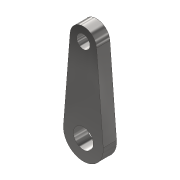
# Autodesk Inventor part: Eslabón 2
Saved by Autodesk Inventor 2021 (Build 250183000, 183)
## iProperties
Created: 2021-10-18
Part Number: Eslabón 2
Material: Stainless Steel
Document SubType Name: Modeling
Designer: Usuario
Density: 8 g/cm^3
Appearance: Semi-Polished
Author: Usuario
Autodesk Inventor part; units mm, degrees
ref_plane "YZ Plane" through (0, 0, 0) normal (1, 0, 0) x (0, 1, 0)
ref_plane "XZ Plane" through (0, 0, 0) normal (0, 1, 0) x (-1, 0, 0)
ref_plane "XY Plane" through (0, 0, 0) normal (0, 0, 1) x (1, 0, 0)
sketch "Sketch1" plane through (0, 0, 0) normal (0, 0, 1) x (1, 0, 0)
  circle A0 centre (0, 0) radius 7.5
  circle A1 centre (0, 63) radius 5
  circle A2 centre (0, 0) radius 15
  circle A3 centre (0, 63) radius 10
  line L0 (-9.9685, 63.7937) -> (-14.9527, 1.1905)
  line L1 (9.9685, 63.7937) -> (14.9527, 1.1905)
  dimension "d0" = 63
  dimension "d1" = 30
  dimension "d2" = 20
  dimension "d3" = 10
  dimension "d4" = 15
  constraints: 4 centre point, 4 end point, 4 point on circle, 4 tangent, 3 coincident
  measures "d0" distance of point (0, 0) A1.centre
  measures "d1" diameter of A2
  measures "d2" diameter of A3
  measures "d3" diameter of A1
  measures "d4" diameter of A0
extrude "Extrusion1" add sketch "Sketch1" along normal mid plane 10
body "Solid1"
